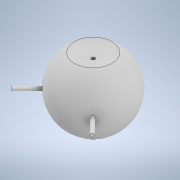
# Autodesk Inventor part: solid mid ball
Saved by Autodesk Inventor 2022 (Build 260153000, 153)
## iProperties
Created: 2022-03-15
Part Number: solid mid ball
Material: Generic
Document SubType Name: Modeling
Designer: mogje
Density: 1 g/cm^3
Appearance: Default
Author: mogje
Autodesk Inventor part; units mm, degrees
ref_plane "YZ Plane" through (0, 0, 0) normal (1, 0, 0) x (0, 1, 0)
ref_plane "XZ Plane" through (0, 0, 0) normal (0, 1, 0) x (-1, 0, 0)
ref_plane "XY Plane" through (0, 0, 0) normal (0, 0, 1) x (1, 0, 0)
sketch "Sketch3" plane through (0, 0, 0) normal (1, 0, 0) x (0, 1, 0)
  line L0 (-27.1198, 0) -> (-27.1198, -16.51)
  line L1 (27.1198, 0) -> (27.1198, -16.51)
  arc A0 (-27.1198, -16.51) -> (27.1198, -16.51) centre (0, 0) ccw
  line L2 (27.1198, 0) -> (-27.1198, 0)
  constraints: 6 end point, 2 point on circle, 2 vertical, 1 centre point, 1 coincident
revolve "Revolution2" add sketch "Sketch3" angle 360 about axis through (0, 27.1198, 0) along (0, -1, 0)
sketch "Sketch5" plane through (0, 27.1198, 0) normal (0, 1, 0) x (1, 0, 0)
  circle A0 centre (0, 0) radius 1.5875
  dimension "d7" = 3.175
  constraints: 1 centre point, 1 coincident
  measures "d7" diameter of A0
extrude "Extrusion1" cut sketch "Sketch5" against normal blind 23.6728
sketch "Sketch6" plane through (0, 0, 0) normal (1, 0, 0) x (0, 1, 0)
  line L0 (27.1198, 16.51) -> (27.1198, -16.51) projected
  line L1 (27.1198, 16.51) -> (54.2396, 0)
  line L2 (54.2396, 0) -> (27.1198, -16.51)
  line L3 (27.1198, 16.51) -> (27.1198, -16.51)
  arc A0 (22.4896, 0) -> (27.1198, -16.51) centre (54.2396, 0) ccw
  line L4 (85.9896, 0) -> (22.4896, 0)
  point P0 (0, 0)
  point P1 (27.1198, 0)
  dimension "d10" = 31.75
  dimension "d11" = 31.75
  dimension "d12" = 33.02
  dimension "d13" = 63.5
  constraints: 8 end point, 2 point on circle, 1 centre point, 1 coincident, 1 collinear, 1 point on line
  measures "d10" distance of L0.start L1.end
  measures "d11" distance of L0.end L1.end
  measures "d12" distance of L3.start L0.end
  measures "d13" distance of L4.end L4.start
revolve "Revolution3" cut sketch "Sketch6" angle 360 about axis through (0, 85.9896, 0) along (0, -1, 0) contours L0 A0 L4
sketch "Sketch7" plane through (0, -27.1198, 0) normal (0, -1, 0) x (1, 0, 0)
  circle A0 centre (0, 0) radius 1.5875 projected
  circle A1 centre (0, 0) radius 1.5875
  point P0 (0, 0)
  constraints: 1 centre point, 1 coincident
extrude "Extrusion2" cut sketch "Sketch7" against normal blind 23.6728
sketch "Sketch8" plane through (0, 0, 0) normal (1, 0, 0) x (0, 1, 0)
  line L0 (-27.1198, 16.51) -> (-27.1198, -16.51) projected
  line L1 (-27.1198, 16.51) -> (-27.1198, -16.51)
  line L2 (-27.1198, -16.51) -> (-54.2396, 0)
  line L3 (-54.2396, 0) -> (-27.1198, 16.51)
  circle A0 centre (-54.2396, 0) radius 31.75
  line L4 (-54.2396, 0) -> (-22.4896, 0)
  point P0 (0, 0)
  point P1 (-27.1198, 0)
  point P2 (-22.4896, 0)
  dimension "d17" = 33.02
  dimension "d18" = 31.75
  dimension "d19" = 31.75
  dimension "d20" = 31.75
  constraints: 8 end point, 1 coincident, 1 collinear, 1 horizontal, 3 other
  measures "d17" distance of L0.start L0.end
  measures "d18" distance of L0.end L2.end
  measures "d19" distance of L0.start L2.end
  measures "d20" distance of L4.start L4.end
revolve "Revolution4" cut sketch "Sketch8" angle 360 about axis through (0, -54.2396, 0) along (0, 1, 0) picked at (-26.272, 9.2768) contours A0 L4 L0
sketch "Sketch9" plane through (0, 0, 0) normal (0, 1, 0) x (-1, 0, 0)
  circle A0 centre (0, 0) radius 31.75
  line L0 (30.7725, 7.8175) -> (7.1862, 30.9261)
  line L1 (-30.7725, 7.8175) -> (-7.1862, 30.9261)
  constraints: 4 end point, 1 centre point
extrude "Extrusion3" cut sketch "Sketch9" along normal mid plane 101.6 contours A0 L1 L0 keep common part
sketch "Sketch10" plane through (18.9794, 0, 19.3718) normal (0.6998, 0, 0.7143) x (0.7143, 0, -0.6998)
  circle A0 centre (0, 0) radius 1.5875
  dimension "d24" = 3.175
  constraints: 1 centre point, 1 coincident
  measures "d24" diameter of A0
extrude "Extrusion4" add sketch "Sketch10" along normal blind 23.6728
sketch "Sketch11" plane through (-18.9794, 0, 19.3718) normal (-0.6998, 0, 0.7143) x (0.7143, 0, 0.6998)
  circle A0 centre (0, 0) radius 1.5875
  dimension "d27" = 3.175
  constraints: 1 centre point, 1 coincident
  measures "d27" diameter of A0
extrude "Extrusion5" add sketch "Sketch11" along normal blind 23.6728
sketch "Sketch12" plane through (0, 0, 0) normal (0, 1, 0) x (-1, 0, 0)
  circle A0 centre (0, 0) radius 1.5875 projected
  circle A1 centre (0, 0) radius 31.75
  arc A2 (-30.7725, 7.8175) -> (-7.1862, 30.9261) centre (0, 0) ccw projected
  line L0 (-31.75, 0) -> (31.75, 0)
  point P0 (-1.5875, 0)
  point P1 (1.5875, 0)
  point P2 (31.75, 0)
  constraints: 2 end point, 2 point on circle, 1 centre point, 1 coincident, 1 horizontal
revolve "Revolution5" add sketch "Sketch12" angle 110 mid plane about axis through (31.75, 0, 0) along (-1, 0, 0) picked at (21.4293, 2.3601) contours A0 L0 A1
body "Solid2"
